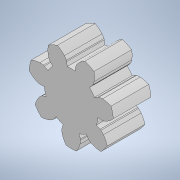
# Autodesk Inventor part: 初段多段部分歯数7
Saved by Autodesk Inventor 2022.2 (Build 262287030, 287C)
## iProperties
Created: 2022-02-22
Part Number: 初段多段部分歯数7
Material: Generic
Document SubType Name: Modeling
Designer: acps
Density: 1 g/cm^3
Appearance: Default
Author: acps
Autodesk Inventor part; units mm, degrees
ref_plane "YZ Plane" through (0, 0, 0) normal (1, 0, 0) x (0, 1, 0)
ref_plane "XZ Plane" through (0, 0, 0) normal (0, 1, 0) x (-1, 0, 0)
ref_plane "XY Plane" through (0, 0, 0) normal (0, 0, 1) x (1, 0, 0)
sketch "Sketch1" plane through (0, 0, 0) normal (0, 0, 1) x (1, 0, 0)
  arc A0 (0.5156, 3.3554) -> (0.4821, 3.2534) centre (0.9432, 3.1583) ccw
  arc A1 (0.7215, 3.6793) -> (0.5156, 3.3554) centre (1.7274, 2.8124) ccw
  arc A2 (1.4571, 4.2576) -> (0.7215, 3.6793) centre (2.5636, 2.0932) ccw
  arc A3 (-2.3019, 2.4952) -> (-2.2431, 2.4054) centre (-1.8812, 2.7066) ccw
  arc A4 (-2.4267, 2.8581) -> (-2.3019, 2.4952) centre (-1.1218, 3.104) ccw
  arc A5 (-2.4202, 3.7937) -> (-2.4267, 2.8581) centre (-0.0382, 3.3094) ccw
  arc A6 (-3.386, -0.244) -> (-3.2791, -0.254) centre (-3.289, 0.2168) ccw
  arc A7 (-3.7476, -0.1153) -> (-3.386, -0.244) centre (-3.1262, 1.0583) ccw
  arc A8 (-4.4751, 0.4731) -> (-3.7476, -0.1153) centre (-2.6112, 2.0335) ccw
  arc A9 (-1.9204, -2.7994) -> (-1.8459, -2.7221) centre (-2.2201, -2.4363) ccw
  arc A10 (-2.2464, -3.0019) -> (-1.9204, -2.7994) centre (-2.7766, -1.7844) ccw
  arc A11 (-3.1601, -3.2037) -> (-2.2464, -3.0019) centre (-3.2179, -0.7736) ccw
  arc A12 (0.9913, -3.2468) -> (0.9773, -3.1404) centre (0.5205, -3.2548) ccw
  arc A13 (0.9463, -3.628) -> (0.9913, -3.2468) centre (-0.3361, -3.2833) ccw
  arc A14 (0.5345, -4.4681) -> (0.9463, -3.628) centre (-1.4015, -2.9982) ccw
  arc A15 (3.1566, -1.2493) -> (3.0646, -1.1939) centre (2.8692, -1.6223) ccw
  arc A16 (3.4265, -1.5221) -> (3.1566, -1.2493) centre (2.3575, -2.3099) ccw
  arc A17 (3.8266, -2.3679) -> (3.4265, -1.5221) centre (1.4703, -2.9651) ccw
  arc A18 (2.9448, 1.689) -> (2.8442, 1.6516) centre (3.0573, 1.2317) ccw
  arc A19 (3.3264, 1.7299) -> (2.9448, 1.689) centre (3.2758, 0.4029) ccw
  arc A20 (4.2372, 1.5154) -> (3.3264, 1.7299) centre (3.2349, -0.6992) ccw
  arc A21 (-0.4821, 3.2534) -> (-0.5156, 3.3554) centre (-0.9432, 3.1583) ccw
  arc A22 (-0.5156, 3.3554) -> (-0.7215, 3.6793) centre (-1.7274, 2.8124) ccw
  arc A23 (-0.7215, 3.6793) -> (-1.4571, 4.2576) centre (-2.5636, 2.0932) ccw
  arc A24 (-2.8442, 1.6516) -> (-2.9448, 1.689) centre (-3.0573, 1.2317) ccw
  arc A25 (-2.9448, 1.689) -> (-3.3264, 1.7299) centre (-3.2758, 0.4029) ccw
  arc A26 (-3.3264, 1.7299) -> (-4.2372, 1.5154) centre (-3.2349, -0.6992) ccw
  arc A27 (-3.0646, -1.1939) -> (-3.1566, -1.2493) centre (-2.8692, -1.6223) ccw
  arc A28 (-3.1566, -1.2493) -> (-3.4265, -1.5221) centre (-2.3575, -2.3099) ccw
  arc A29 (-3.4265, -1.5221) -> (-3.8266, -2.3679) centre (-1.4703, -2.9651) ccw
  arc A30 (-0.9773, -3.1404) -> (-0.9913, -3.2468) centre (-0.5205, -3.2548) ccw
  arc A31 (-0.9913, -3.2468) -> (-0.9463, -3.628) centre (0.3361, -3.2833) ccw
  arc A32 (-0.9463, -3.628) -> (-0.5345, -4.4681) centre (1.4015, -2.9982) ccw
  arc A33 (1.8459, -2.7221) -> (1.9204, -2.7994) centre (2.2201, -2.4363) ccw
  arc A34 (1.9204, -2.7994) -> (2.2464, -3.0019) centre (2.7766, -1.7844) ccw
  arc A35 (2.2464, -3.0019) -> (3.1601, -3.2037) centre (3.2179, -0.7736) ccw
  arc A36 (3.2791, -0.254) -> (3.386, -0.244) centre (3.289, 0.2168) ccw
  arc A37 (3.386, -0.244) -> (3.7476, -0.1153) centre (3.1262, 1.0583) ccw
  arc A38 (3.7476, -0.1153) -> (4.4751, 0.4731) centre (2.6112, 2.0335) ccw
  arc A39 (2.2431, 2.4054) -> (2.3019, 2.4952) centre (1.8812, 2.7066) ccw
  arc A40 (2.3019, 2.4952) -> (2.4267, 2.8581) centre (1.1218, 3.104) ccw
  arc A41 (2.4267, 2.8581) -> (2.4202, 3.7937) centre (0.0382, 3.3094) ccw
  arc A42 (0.4177, 2.8192) -> (-0.4177, 2.8192) centre (0, 0) ccw
  arc A43 (-1.9437, 2.0843) -> (-2.4646, 1.4312) centre (0, 0) ccw
  arc A44 (-2.8415, -0.2201) -> (-2.6556, -1.0346) centre (0, 0) ccw
  arc A45 (-1.5996, -2.3588) -> (-0.8469, -2.7213) centre (0, 0) ccw
  arc A46 (0.8469, -2.7213) -> (1.5996, -2.3588) centre (0, 0) ccw
  arc A47 (2.6556, -1.0346) -> (2.8415, -0.2201) centre (0, 0) ccw
  arc A48 (2.4646, 1.4312) -> (1.9437, 2.0843) centre (0, 0) ccw
  arc A49 (-1.4571, 4.2576) -> (-2.4202, 3.7937) centre (0, 0) ccw
  arc A50 (-4.2372, 1.5154) -> (-4.4751, 0.4731) centre (0, 0) ccw
  arc A51 (-3.8266, -2.3679) -> (-3.1601, -3.2037) centre (0, 0) ccw
  arc A52 (-0.5345, -4.4681) -> (0.5345, -4.4681) centre (0, 0) ccw
  arc A53 (3.1601, -3.2037) -> (3.8266, -2.3679) centre (0, 0) ccw
  arc A54 (4.4751, 0.4731) -> (4.2372, 1.5154) centre (0, 0) ccw
  arc A55 (2.4202, 3.7937) -> (1.4571, 4.2576) centre (0, 0) ccw
  line L0 (0.4177, 2.8192) -> (0.4821, 3.2534)
  line L1 (-1.9437, 2.0843) -> (-2.2431, 2.4054)
  line L2 (-2.8415, -0.2201) -> (-3.2791, -0.254)
  line L3 (-1.5996, -2.3588) -> (-1.8459, -2.7221)
  line L4 (0.8469, -2.7213) -> (0.9773, -3.1404)
  line L5 (2.6556, -1.0346) -> (3.0646, -1.1939)
  line L6 (2.4646, 1.4312) -> (2.8442, 1.6516)
  line L7 (-0.4177, 2.8192) -> (-0.4821, 3.2534)
  line L8 (-2.4646, 1.4312) -> (-2.8442, 1.6516)
  line L9 (-2.6556, -1.0346) -> (-3.0646, -1.1939)
  line L10 (-0.8469, -2.7213) -> (-0.9773, -3.1404)
  line L11 (1.5996, -2.3588) -> (1.8459, -2.7221)
  line L12 (2.8415, -0.2201) -> (3.2791, -0.254)
  line L13 (1.9437, 2.0843) -> (2.2431, 2.4054)
  constraints: 112 point on circle, 56 centre point, 28 end point
extrude "Extrusion1" add sketch "Sketch1" against normal blind 4
body "Solid1"
